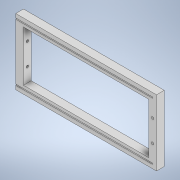
# Autodesk Inventor part: 2020-04-11 CubeBaseSkeleton
Saved by Autodesk Inventor 2020 (Build 240168000, 168)
## iProperties
Created: 2019-12-01
Part Number: 2020-04-11 CubeBaseSkeleton
Material: Generic
Document SubType Name: Modeling
Designer: torto
Density: 1 g/cm^3
Appearance: Default
length: 230.251 mm
height: 107.950 mm
d3: 6.350 mm
d4: 6.350 mm
d5: 223.901 mm
d6: 1.524 mm
spacing: 35.983 mm
d9: 6.350 mm
d10: 3.500 mm
d11: 2.000 ul
d13: 35.983 mm
thickness: 12.700 mm
d19: 0.00 deg
d21: 6.350 mm
d22: 6.350 mm
d23: 223.901 mm
d24: 1.524 mm
d25: 6.350 mm
d26: 0.00 deg
d33: 6.350 mm
d34: 35.983 mm
ScrewDiameter: 4.000 mm
d36: 6.350 mm
d37: 35.983 mm
d38: 4.000 mm
d39: 12.700 mm
d40: 0.00 deg
LcdFrameHoleDiameter: 3.000 mm
InputHoleSpacing: 0.172 in
d80: 0.278 in
InputScrewDiameter: 3.500 mm
d82: 14.100 mm
d83: 8.500 mm
InputHoleSpacingX: 7.100 mm
InputHoleSpacingY: 4.250 mm
ScrewDiameterUntapped: 4.000 mm
ScrewCapDiameter: 3.500 mm
PcbThickness: 1.651 mm
TopScrewDiameter: 4.000 mm
InputScrewDiameterUntapped: 2.500 mm
LeftInputHoleSpacingX: 7.100 mm
Author: torto
Autodesk Inventor part; units mm, degrees
ref_plane "YZ Plane" through (0, 0, 0) normal (1, 0, 0) x (0, 1, 0)
ref_plane "XZ Plane" through (0, 0, 0) normal (0, 1, 0) x (-1, 0, 0)
ref_plane "XY Plane" through (0, 0, 0) normal (0, 0, 1) x (1, 0, 0)
sketch "Sketch1" plane through (0, 0, 0) normal (0, 0, 1) x (1, 0, 0)
  line L0 (0, 0) -> (230.251, 0)
  line L1 (230.251, 0) -> (230.251, 107.95)
  line L2 (230.251, 107.95) -> (0, 107.95)
  line L3 (0, 107.95) -> (0, 0)
  line L4 (230.251, 107.95) -> (223.901, 107.95) construction
  line L5 (223.901, 107.95) -> (223.901, 101.6) construction
  line L6 (223.901, 101.6) -> (230.251, 101.6) construction
  line L7 (230.251, 101.6) -> (230.251, 107.95) construction
  line L8 (223.901, 101.6) -> (0, 101.6)
  line L9 (0, 101.6) -> (0, 100.076)
  line L10 (0, 100.076) -> (223.901, 100.076)
  line L11 (223.901, 100.076) -> (223.901, 101.6)
  line L12 (230.251, 0) -> (223.901, 0) construction
  line L13 (223.901, 0) -> (223.901, 35.9833) construction
  line L14 (223.901, 35.9833) -> (230.251, 35.9833) construction
  line L15 (230.251, 35.9833) -> (230.251, 0) construction
  circle A0 centre (223.901, 35.9833) radius 2
  circle A1 centre (223.901, 71.9667) radius 2
  line L16 (230.251, 53.975) -> (0, 53.975) construction
  line L17 (223.901, 6.35) -> (0, 6.35)
  line L18 (0, 7.874) -> (223.901, 7.874)
  line L19 (223.901, 7.874) -> (223.901, 6.35)
  dimension "length" = 230.251
  dimension "height" = 107.95
  dimension "d3" = 6.35
  dimension "d4" = 6.35
  dimension "d5" = 223.901
  dimension "d6" = 1.524
  dimension "spacing" = 35.9833
  dimension "d9" = 6.35
  dimension "TopScrewDiameter" = 4
  dimension "d13" = 35.9833
  constraints: 40 end point, 8 parallel, 4 horizontal, 4 perpendicular, 4 symmetric about line, 2 centre point, 2 coincident, 2 midpoint, 1 vertical, 3 other
  measures "length" distance of L2.end L1.end
  measures "height" distance of L1.end L0.end
  measures "d3" distance of L5.end L4.end
  measures "d4" distance of L5.end L6.end
  measures "d5" distance of L10.end L9.end
  measures "d6" distance of L9.end L8.end
  measures "spacing" distance of L12.end L13.end
  measures "d9" distance of L13.end L14.end
  measures "TopScrewDiameter" diameter of A0
  measures "d13" distance of A0.centre A1.centre
extrude "Generic Shape" add sketch "Sketch1" along normal blind 12.7
sketch "ScrewCapDiameter" plane through (0, 0, 0) normal (0, 0, -1) x (-1, 0, 0)
  circle A0 centre (-223.901, 71.9667) radius 2 projected
  circle A1 centre (-223.901, 71.9667) radius 4
  circle A2 centre (-223.901, 35.9833) radius 2 projected
  circle A3 centre (-223.901, 35.9833) radius 4
  point P0 (0, 0)
  dimension "d106" = 8
  dimension "d107" = 8
  constraints: 2 centre point, 2 coincident
  measures "d106" diameter of A1
  measures "d107" diameter of A3
extrude "ScrewCapCountersink" cut sketch "ScrewCapDiameter" against normal blind 4
sketch "PcbNotchDimensions" plane through (0, 0, 12.7) normal (0, 0, 1) x (1, 0, 0)
  line L0 (230.251, 107.95) -> (0, 107.95) construction
  line L1 (230.251, 107.95) -> (223.901, 107.95) construction
  line L2 (223.901, 107.95) -> (223.901, 101.6) construction
  line L3 (223.901, 101.6) -> (230.251, 101.6) construction
  line L4 (230.251, 101.6) -> (230.251, 107.95) construction
  line L5 (223.901, 101.6) -> (0, 101.6)
  line L6 (0, 101.6) -> (0, 99.949)
  line L7 (0, 99.949) -> (223.901, 99.949)
  line L8 (223.901, 99.949) -> (223.901, 101.6)
  line L9 (230.251, 0) -> (230.251, 107.95) construction
  line L10 (230.251, 53.975) -> (0, 53.975) construction
  line L11 (0, 107.95) -> (0, 0) construction
  line L12 (223.901, 6.35) -> (0, 6.35)
  line L13 (0, 6.35) -> (0, 8.001)
  line L14 (0, 8.001) -> (223.901, 8.001)
  line L15 (223.901, 8.001) -> (223.901, 6.35)
  point P0 (230.251, 106.45)
  point P1 (0, 106.45)
  dimension "d21" = 6.35
  dimension "d22" = 6.35
  dimension "d23" = 223.901
  dimension "PcbThickness" = 1.651
  constraints: 26 end point, 4 parallel, 4 symmetric about line, 2 horizontal, 2 midpoint, 2 perpendicular
  measures "d21" distance of L2.end L1.end
  measures "d22" distance of L2.end L3.end
  measures "d23" distance of L7.end L6.end
  measures "PcbThickness" distance of L6.end L5.end
extrude "PCB Notch" cut sketch "PcbNotchDimensions" against normal blind 6.35
sketch "UntappedScrewHoleDimensions" plane through (0, 0, 0) normal (-1, 0, 0) x (0, 0, 1)
  line L0 (0, 0) -> (6.35, 0) construction
  line L1 (6.35, 0) -> (6.35, 35.9833) construction
  line L2 (6.35, 35.9833) -> (0, 35.9833) construction
  line L3 (0, 35.9833) -> (0, 0) construction
  circle A0 centre (6.35, 35.9833) radius 2
  line L4 (0, 107.95) -> (6.35, 107.95) construction
  line L5 (6.35, 107.95) -> (6.35, 71.9667) construction
  line L6 (6.35, 71.9667) -> (0, 71.9667) construction
  line L7 (0, 71.9667) -> (0, 107.95) construction
  circle A1 centre (6.35, 71.9667) radius 2
  dimension "d33" = 6.35
  dimension "d34" = 35.9833
  dimension "ScrewDiameterUntapped" = 4
  dimension "d36" = 6.35
  dimension "d37" = 35.9833
  dimension "d38" = 4
  constraints: 16 end point, 4 parallel, 2 centre point, 2 coincident, 2 horizontal, 2 perpendicular
  measures "d33" distance of L2.end L1.end
  measures "d34" distance of L1.end L0.end
  measures "ScrewDiameterUntapped" diameter of A0
  measures "d36" distance of L5.end L6.end
  measures "d37" distance of L4.end L5.end
  measures "d38" diameter of A1
extrude "UntappedScrewDepth" cut sketch "UntappedScrewHoleDimensions" against normal blind 12.7
thread "Thread10" size "M4x0.7" class "6H" standard "ANSI Metric M Profile" length 230.251
thread "Thread11" size "M4x0.7" class "6H" standard "ANSI Metric M Profile" length 230.251
sketch "Sketch18" plane through (0, 0, 0) normal (0, 0, -1) x (-1, 0, 0)
  line L0 (0, 0) -> (-12.7, 0) construction
  line L1 (-12.7, 0) -> (-12.7, 12.7) construction
  line L2 (-12.7, 12.7) -> (0, 12.7) construction
  line L3 (0, 12.7) -> (0, 0) construction
  line L4 (-12.7, 12.7) -> (-217.551, 12.7)
  line L5 (-217.551, 12.7) -> (-217.551, 95.25)
  line L6 (-217.551, 95.25) -> (-12.7, 95.25)
  line L7 (-12.7, 95.25) -> (-12.7, 12.7)
  dimension "bezel" = 12.7
  dimension "d156" = 12.7
  dimension "d157" = 204.851
  dimension "d158" = 82.55
  constraints: 16 end point, 4 parallel, 2 horizontal, 2 perpendicular
  measures "bezel" distance of L1.end L2.end
  measures "d156" distance of L0.end L1.end
  measures "d157" distance of L5.end L6.end
  measures "d158" distance of L4.end L5.end
extrude "Extrusion16" cut sketch "Sketch18" against normal blind 12.7
equation "\"d3\" = 0.5 * thickness"
equation "\"d4\" = 0.5 * thickness"
equation "\"d5\" = length - 0.5 * thickness"
equation "\"spacing\" = 0.333333 * height"
equation "\"d9\" = 0.5 * thickness"
equation "\"d13\" = spacing"
equation "\"d25\" = 0.5 * thickness"
equation "\"d33\" = 0.5 * thickness"
equation "\"d34\" = 0.333333 * height"
equation "\"d36\" = 0.5 * thickness"
equation "\"d37\" = 0.333333 * height"
equation "\"d38\" = ScrewDiameterUntapped"
equation "\"LcdThickness\" = 9.9"
equation "\"thickness\" = 12.7"
body "Solid1"
